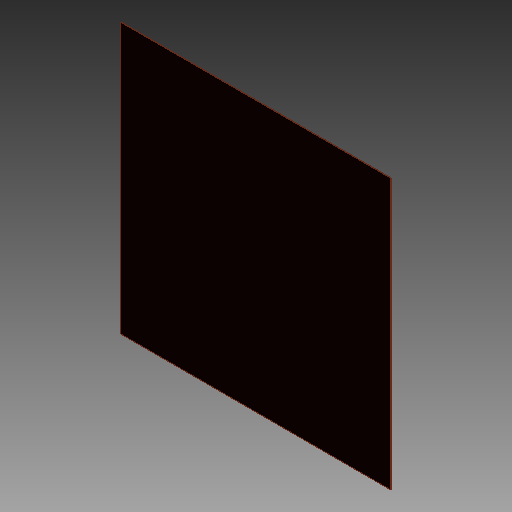
# Autodesk Inventor part: 2221_Copper Box Side_V1
Saved by Autodesk Inventor 2020 (Build 240168000, 168)
## iProperties
Created: 2017-08-01
Part Number: 2221_Copper Box Side_V1
Material: Copper
Document SubType Name: Modeling
Designer: MPI
Density: 8.94 g/cm^3
Appearance: Copper - Satin
Mass: 3544.14 g
Surface Area: 7458.26 cm^2
Volume: 396.436 cm^3
Author: MPI
Autodesk Inventor part; units mm, degrees
ref_plane "YZ Plane" through (0, 0, 0) normal (1, 0, 0) x (0, 1, 0)
ref_plane "XZ Plane" through (0, 0, 0) normal (0, 1, 0) x (-1, 0, 0)
ref_plane "XY Plane" through (0, 0, 0) normal (0, 0, 1) x (1, 0, 0)
sketch "Sketch1" plane through (0, 0, 0) normal (0, 0, 1) x (1, 0, 0)
  line L0 (-304.8, -304.8) -> (304.8, -304.8)
  line L1 (304.8, -304.8) -> (304.8, 304.8)
  line L2 (304.8, 304.8) -> (-304.8, 304.8)
  line L3 (-304.8, 304.8) -> (-304.8, -304.8)
  line L4 (-304.8, -304.8) -> (304.8, 304.8) construction
  line L5 (304.8, -304.8) -> (-304.8, 304.8) construction
  point P0 (0, 0)
  dimension "d0" = 609.6
  dimension "d1" = 609.6
  constraints: 12 end point, 2 midpoint, 2 parallel, 1 horizontal, 1 perpendicular
  measures "d0" distance of L2.end L1.end
  measures "d1" distance of L1.end L0.end
extrude "Extrusion1" add sketch "Sketch1" along normal blind 1.0668
body "Solid1"
